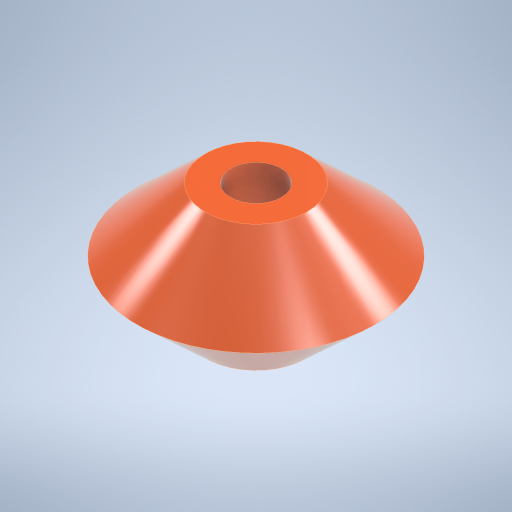
# Autodesk Inventor part: soroban_sep
Saved by Autodesk Inventor 2023 (Build 270158000, 158)
## iProperties
Created: 2023-04-24
Part Number: soroban_sep
Material: 一般
Document SubType Name: Modeling
Designer: zegi
Density: 1 g/cm^3
Appearance: 滑らか - 淡いオレンジ
Author: zegi
Autodesk Inventor part; units mm, degrees
ref_plane "YZ Plane" through (0, 0, 0) normal (1, 0, 0) x (0, 1, 0)
ref_plane "XZ Plane" through (0, 0, 0) normal (0, 1, 0) x (-1, 0, 0)
ref_plane "XY Plane" through (0, 0, 0) normal (0, 0, 1) x (1, 0, 0)
sketch "スケッチ1" plane through (0, 0, 0) normal (0, 0, 1) x (1, 0, 0)
  line L0 (0, 3.75) -> (3, 3.75)
  line L1 (0, -3.75) -> (3, -3.75)
  line L2 (0, 0) -> (7.05, 0)
  line L3 (0, 3.75) -> (0, -3.75)
  line L4 (3, -3.75) -> (7.05, 0)
  line L5 (3, 3.75) -> (7.05, 0)
  line L6 (0, -5.25) -> (0, 5.25) projected
  line L7 (1.5, 3.75) -> (1.5, -3.75)
  dimension "d1" = 7.5
  dimension "d2" = 7.05
  dimension "d3" = 3
  dimension "d5" = 1.5
  constraints: 14 end point, 3 horizontal, 2 midpoint, 2 vertical, 2 vertical alignment, 1 parallel, 1 other
  measures "d1" distance between parallel lines of L1 L0
  measures "d2" distance of L2.start L2.end
  measures "d3" distance of L0.start L0.end
  measures "d5" distance between parallel lines of L3 L7
revolve "回転1" add sketch "スケッチ1" angle 360 about axis through (0, -10, 0) along (0, 1, 0) contours L0 L5 L2 L7 | L2 L4 L1 L7
